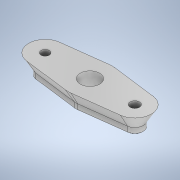
# Autodesk Inventor part: Practica4
Saved by Autodesk Inventor 2020 (Build 240168000, 168)
## iProperties
Created: 2020-02-12
Part Number: Practica4
Material: Aluminio 6061-AHC
Document SubType Name: Chapa
Designer: luisg
Density: 2.7 g/cm^3
Sheet Metal Rule: Por defecto_mm
Appearance: Aluminio - Oscuro
Author: luisg
Autodesk Inventor part; units mm, degrees
ref_plane "YZ Plane" through (0, 0, 0) normal (1, 0, 0) x (0, 1, 0)
ref_plane "XZ Plane" through (0, 0, 0) normal (0, 1, 0) x (-1, 0, 0)
ref_plane "XY Plane" through (0, 0, 0) normal (0, 0, 1) x (1, 0, 0)
sketch "Boceto1" plane through (0, 0, 0) normal (0, 1, 0) x (-1, 0, 0)
  arc A0 (81.875, -14.8824) -> (81.875, 14.8824) centre (80, 0) ccw
  line L0 (81.875, -14.8824) -> (3.125, -24.8039)
  line L1 (3.125, 24.8039) -> (81.875, 14.8824)
  line L2 (0, -32.0701) -> (0, 49.2426) construction
  arc A1 (-81.875, 14.8824) -> (-81.875, -14.8824) centre (-80, 0) ccw
  line L3 (-81.875, -14.8824) -> (-3.125, -24.8039)
  line L4 (-3.125, 24.8039) -> (-81.875, 14.8824)
  arc A2 (3.125, 24.8039) -> (-3.125, 24.8039) centre (0, 0) ccw
  arc A3 (-3.125, -24.8039) -> (3.125, -24.8039) centre (0, 0) ccw
  dimension "d1" = 30
  dimension "d2" = 80
  constraints: 10 end point, 8 point on circle, 5 symmetric about line, 4 centre point, 4 tangent, 1 coincident, 1 vertical, 1 other
  measures "d1" diameter of A0
  measures "d2" distance of point (0, 0) A0.centre
extrude "Extrusión1" add sketch "Boceto1" along normal blind 25 draft 30 and the other way blind 10
sketch "Boceto2" plane through (0, -10, 0) normal (0, -1, 0) x (1, 0, 0)
  arc A0 (81.875, -14.8824) -> (81.875, 14.8824) centre (80, 0) ccw projected
  line L0 (81.875, 14.8824) -> (3.125, 24.8039) projected
  arc A1 (3.125, 24.8039) -> (-3.125, 24.8039) centre (0, 0) ccw projected
  line L1 (-3.125, 24.8039) -> (-81.875, 14.8824) projected
  arc A2 (-81.875, 14.8824) -> (-81.875, -14.8824) centre (-80, 0) ccw projected
  line L2 (-81.875, -14.8824) -> (-3.125, -24.8039) projected
  arc A3 (-3.125, -24.8039) -> (3.125, -24.8039) centre (0, 0) ccw projected
  line L3 (3.125, -24.8039) -> (81.875, -14.8824) projected
  circle A4 centre (0, 0) radius 17.1981
  circle A5 centre (-80, 0) radius 7.3963
  circle A6 centre (80, 0) radius 8.3739
  constraints: 3 centre point, 3 coincident
extrude "Extrusión2" cut sketch "Boceto2" against normal through all contours A4 | A5 | A6
chamfer "Chaflán1" distance 2 angle 45 1 edges at (-87.3963, -10, 0)
chamfer "Chaflán2" distance 2 angle 45 1 edges at (-17.1981, -10, 0)
chamfer "Chaflán3" distance 2 angle 45 1 edges at (71.6261, -10, 0)
fillet "Empalme1" radius 1 8 edges at (0, -10, -25) (42.5, -10, -19.8431) (95, -10, 0) (42.5, -10, 19.8431) (0, -10, 25) (-42.5, -10, 19.8431) (-95, -10, 0) (-42.5, -10, -19.8431)
equation "\"Radio_pliegue\" = Grosor"
equation "\"Anchura_desahogo_plegado\" = Grosor"
equation "\"Profundidad_desahogo_plegado\" = 0.5 * Grosor"
equation "\"Tamaño_destalonado\" = 4 * Grosor"
equation "\"Remanente_mínimo\" = 2 * Grosor"
equation "\"Radiodetransición\" = Radio_pliegue"
equation "\"Tamaño_de_radio_de_Jacobi\" = Radio_pliegue"
equation "\"TamañoSeparación\" = Grosor"
equation "\"Grosor\" = 0.5"
